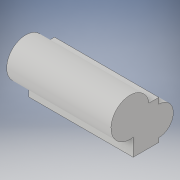
# Autodesk Inventor part: test
Saved by Autodesk Inventor 2017 SP1 (Build 210196100, 196)
## iProperties
Created: 2017-12-20
Part Number: test
Material: Generic
Document SubType Name: Modeling
Designer: User
Density: 1 g/cm^3
Appearance: Default
Author: User
Autodesk Inventor part; units mm, degrees
ref_plane "YZ Plane" through (0, 0, 0) normal (1, 0, 0) x (0, 1, 0)
ref_plane "XZ Plane" through (0, 0, 0) normal (0, 1, 0) x (-1, 0, 0)
ref_plane "XY Plane" through (0, 0, 0) normal (0, 0, 1) x (1, 0, 0)
sketch "Sketch1" plane through (0, 0, 0) normal (1, 0, 0) x (0, 1, 0)
  circle A0 centre (5.3535, -5.8605) radius 7.071
  circle A1 centre (13.9111, 8.1317) radius 9.3306
  line L0 (-3.7313, 6.6311) -> (15.29, 6.6311)
  line L1 (15.29, 6.6311) -> (15.29, -5.8605)
  line L2 (15.29, -5.8605) -> (-3.7313, -5.8605)
  line L3 (-3.7313, -5.8605) -> (-3.7313, 6.6311)
  point P0 (0, 0)
  constraints: 8 end point, 2 centre point, 2 parallel, 1 horizontal, 1 perpendicular, 1 tangent
extrude "Extrusion1" add sketch "Sketch1" along normal blind 50.8
body "Solid1"
